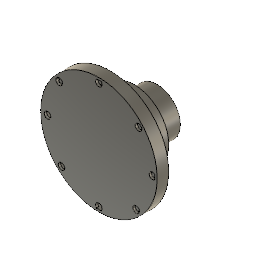
_Coupling Flange.14848507-ee6e-4340-aef8-018ab998a0ea (Autodesk Fusion 360 design; units mm, degrees)
Autodesk Fusion 360 part; units mm, degrees
sketch "Sketch1" plane through (0, 0, 0) normal (0, 1, 0) x (1, 0, 0)
  circle A0 centre (0, 0) radius 25
  circle A1 centre (0.1317, -22.5832) radius 1.214
  circle A2 centre (20, 0) radius 1.7262
extrude "Extrude1" add sketch "Sketch1" along normal blind 5 contours A0 | A1 | A2
sketch "Sketch2" plane through (0, 5, 0) normal (0, 1, 0) x (-1, 0, 0)
  circle A0 centre (0, 0) radius 25
  circle A1 centre (0, 0) radius 20
extrude "Extrude2" add sketch "Sketch2" along normal blind 2 contours A1
sketch "Sketch3" plane through (0, 7, 0) normal (0, 1, 0) x (-1, 0, 0)
  circle A0 centre (0, 0) radius 20
  circle A1 centre (0, 0) radius 15
extrude "Extrude3" add sketch "Sketch3" along normal blind 8 contours A1
sketch "Sketch4" plane through (0, 15, 0) normal (0, 1, 0) x (-1, 0, 0)
  circle A0 centre (0, 0) radius 15
  circle A1 centre (0, 0) radius 10
extrude "Extrude4" add sketch "Sketch4" along normal blind 10 contours A1
shell "Shell1" thickness 1 removed faces 1 at (-2.3712, 25, -3.5556)
sketch "Sketch5" plane through (0, 5, 0) normal (0, 1, 0) x (-1, 0, 0)
  circle A0 centre (0, 0) radius 20
  circle A1 centre (0, 0) radius 25
  circle A2 centre (0, 23) radius 1.4142
  circle A3 centre (-23, 0) radius 1.414
  circle A4 centre (0, -23) radius 1.414
  circle A5 centre (22, 0) radius 1.414
  circle A6 centre (-17, 15) radius 1.4142
  circle A7 centre (17, 15) radius 1.4
  circle A8 centre (16, -16) radius 1.3726
  circle A9 centre (0, 0) radius 24
  circle A10 centre (-16, -16) radius 1.4142
  line L0 (75, 30) -> (75, -30)
  line L1 (80, 20) -> (80, 0)
  line L2 (80, 0) -> (105, 0)
  line L3 (105, 0) -> (105, 5)
  line L4 (105, 5) -> (90, 5)
  line L5 (90, 5) -> (90, 7)
  line L6 (85, 7) -> (85, 20)
  line L7 (85, 20) -> (80, 20)
  line L8 (85, 7) -> (90, 7)
  dimension "d10" = 2.828
  dimension "d11" = 2.828
  dimension "d12" = 2.828
  dimension "d13" = 2.8
  measures "d10" diameter of A3
  measures "d11" diameter of A4
  measures "d12" diameter of A5
  measures "d13" diameter of A7
extrude "Extrude5" cut sketch "Sketch5" against normal blind 5 contours A2 A9 | A8 | A7 A9 | A6 A9 | A3 A9 | A4 A9 | A9 A10 | A5 picked at (-0.0096, 23.1937) picked at (17.3227, 15.2673) picked at (-17.3125, 15.2713) picked at (-23.1937, 0) picked at (-0.0096, -23.1938) picked at (-16.2973, -16.3307)
